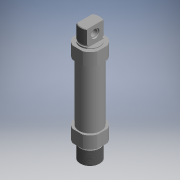
# Autodesk Inventor part: 193992 DSNU-32-60-PPS---(A----0-ZR)
Saved by Autodesk Inventor 2017.3 (Build 213256000, 256)
## iProperties
Part Number: 193992 DSNU-32-60-PPS---(A----0-ZR)
Material: Generic
Catalog Web Link: www.cadenas.de
Description: DSNU---(ZR)-Standard cylinder
Vendor: FESTO
Document SubType Name: Modeling
Designer: partserver
Manufacturer: FESTO
Mass: 95.0969 g
Surface Area: 336.432 cm^2
Volume: 95.0969 cm^3
Density: 1 g/cm^3
Appearance: PSOLRGB-192-192-192
Category: PARTsolutions
Company: FESTO
Title: 193992 DSNU-32-60-PPS
Author: Cadenas PARTsolutions
Comments: Standard cylinder
PSOL_IDENT_0: {$CADENAS_DATA\23d-libs\festo\parts\d\dsnu\parts\dsnu_metric_zr.prj},238 {VTYP=3D},{NB=193992 DSNU-3
PSOL_IDENT_1: 2-60-PPS---(A----0-ZR)},{LINA=193992 DSNU-32-60-PPS},{NN=DSNU---(ZR)},{DATE=25.01.2021 09:43:10},{GE
PSOL_IDENT_2: OMDATE=15.09.2020 12:46:13},{VERSION=},{LINEID=70},{WBVAR=TNR,HUB,DA,PE,ZD,VS,KA,K8,KP,R8},{WBNUMERI
PSOL_IDENT_3: C=HUB,K8}  {NB=193992 DSNU-32-60-PPS---(A----0-ZR)},{LINA=193992 DSNU-32-60-PPS},{KT=DUMMY},{TNR=193
PSOL_IDENT_4: 992},{TYP=DSNU-32},{DSNU=METRIC},{DE=D},{KDM=32},{HUB=60},{DA=PPS},{DA1='P','PPV','PPS'},{PE=A},{ZD=
PSOL_IDENT_5: -},{VS=-},{VSALG='-','Q'},{KA=-},{KAALG='-','S2'},{K8=0},{KP=-},{KPALG='-','KP'},{R8=-},{R81='-','R8'
PSOL_IDENT_6: },{R8H=26.200},{A1=35},{A2=500},{A3=8},{A4=55.5},{AB=30},{AM=22},{B=30},{BB=4},{BE=M30x1,5},{BENDM=3
PSOL_IDENT_7: 0.000},{BEKDM=28.160},{BEP=1.500},{BS=6.6},{B1=48},{B2=10},{B3=30},{B4=9},{B5=25.0},{B6=11},{B7=3},{
PSOL_IDENT_8: CD=10},{D=38},{D1=30},{D2=12},{D3=33.6},{D4=10.0},{D5=34.0},{D6=42},{D7=30},{EE=G1/8},{EENDM=9.7280}
PSOL_IDENT_9: ,{EEKDM=8.5660},{EW=16},{F=38},{FF=M5},{FFNDM=5.000},{FFKDM=4.019},{F1=19},{H=40},{H1=6},{KK=M10x1.2
PSOL_IDENT_10: 5},{KKNDM=10.0000},{KKKDM=8.1600},{KKP=1.250},{K1=M6},{K1NDM=6.000},{K1KDM=4.773},{K2=2.5},{KV=0},{K
PSOL_IDENT_11: W=8},{L=13},{LH=12.0},{LK=15.0},{L1=129.5},{L2=69.5},{L3=9.0},{L4=26.0},{L5=24},{L6=56},{L7=30},{L8=
PSOL_IDENT_12: 19.0},{L9=25.0},{L10=85.5},{L11=97.5},{L12=65.5},{L13=137.5},{ST=6.8},{SW=10},{T=12},{WH=34},{X=2.6}
PSOL_IDENT_13: ,{XC=117.5},{K1KP=46},{K2KP=M5},{K2KPNDM=5.000},{K3KP=12},{K4KP=23.0},{K5KP=67.5},{K6KP=4.4},{K7KP=2
PSOL_IDENT_14: 0},{K8KP=30.0},{K9KP=12.5},{K10KP=5.0},{K11KP=15},{K12KP=M5},{K12KPNDM=5.000},{K13KP=55},{ZRSTART=45
PSOL_IDENT_15: },{MHL=35.000},{ZRL=31.5},{C=17.200},{WHX=12.000},{LD1=27.800},{LD2=27.700},{AD1=11.000},{AD2=8.000}
PSOL_IDENT_16: ,{AD3=8.500},{AD4=7.000},{AD5=10.500},{MH1=11.000},{MH2=2.100},{MH3=15.200},{KP1=25.000},{KP2=26.000
PSOL_IDENT_17: },{KP3=20.000},{KP4=20.000},{KP5=36.000},{KPC=18.000},{KPF=3.000},{KPG=17.500},{KPH=62.000},{KPJ=19.
PSOL_IDENT_18: 500},{KPK=17.000},{KPL=4.500},{KPR3=1.000},{KPR=19.000},{KPS=16.000},{MLD1=45.000},{MLD2=40.000},{ML
PSOL_IDENT_19: D3=5.000},{MLL1=14.000},{PPVSTD=14.500},{PPVMH=28.000},{PPVMQ=4.500},{PPVY=9.000},{PPVZ=12.800},{PPV
PSOL_IDENT_20: A=4.000},{PPVB=0.500},{PPVC=1.000},{PPVD=1.000},{PPVE=8.000},{PPVH=15.000},{KL1=65},{SWL=6.000},{K3L=
PSOL_IDENT_21: 6.400},{ES1=2.500},{ES2=8.500},{KPVERS=0},{HUB1=60},{NUTOFF=8.500},{DIMZJREAR=181.5},{KAVERS=0},{VER
PSOL_IDENT_22: S=2},{H2=38}
NB: 193992 DSNU-32-60-PPS---(A----0-ZR)
NN: DSNU---(ZR)
NT: Standard cylinder
NBSYN: $TNR. $TYP.-$HUB1.-$DA.---($PE.$ZD.$VS.$KA.$KP.$K8.$R8.ZR)
LINA: 193992 DSNU-32-60-PPS
CATALOG: Festo
TNR: 193992
TYP: DSNU-32
DSNU: METRIC
DE: D
KDM: 32
HUB: 60
DA: PPS
DA1: 'P','PPV','PPS'
PE: A
ZD: -
VS: -
KA: -
K8: 0
KP: -
R8: -
R81: '-','R8'
R8H: 26.2
A1: 35
A2: 500
A3: 8
A4: 55.5
AB: 30
AM: 22
B: 30
BB: 4
BE: M30x1,5
BENDM: 30
BEKDM: 28.16
BEP: 1.5
BS: 6.6
B1: 48
B2: 10
B3: 30
B4: 9
B5: 25
B6: 11
B7: 3
CD: 10
D: 38
D1: 30
D2: 12
D3: 33.6
D4: 10
D5: 34
D6: 42
D7: 30
EE: G1/8
EENDM: 9.728
EEKDM: 8.566
EW: 16
F: 38
FF: M5
FFNDM: 5
FFKDM: 4.019
F1: 19
H: 40
H1: 6
KK: M10x1.25
KKNDM: 10
KKKDM: 8.16
KKP: 1.25
K1: M6
K1NDM: 6
K1KDM: 4.773
K2: 2.5
KV: 0
KW: 8
L: 13
LH: 12
LK: 15
L3: 9
L4: 26
L5: 24
L6: 56
L7: 30
L8: 19
L9: 25
L13: 137.5
ST: 6.8
SW: 10
T: 12
X: 2.6
K1KP: 46
K2KP: M5
K2KPNDM: 5
K3KP: 12
K4KP: 23
K5KP: 67.5
K6KP: 4.4
K7KP: 20
K8KP: 30
K9KP: 12.5
K10KP: 5
K11KP: 15
K12KP: M5
K12KPNDM: 5
K13KP: 55
MHL: 35
C: 17.2
WHX: 12
LD1: 27.8
LD2: 27.7
AD1: 11
AD2: 8
AD3: 8.5
AD4: 7
AD5: 10.5
MH1: 11
MH2: 2.1
MH3: 15.2
KP1: 25
KP2: 26
KP3: 20
KP4: 20
KP5: 36
KPC: 18
KPF: 3
KPG: 17.5
KPH: 62
KPJ: 19.5
KPK: 17
KPL: 4.5
KPR3: 1
KPR: 19
KPS: 16
MLD1: 45
MLD2: 40
MLD3: 5
MLL1: 14
PPVSTD: 14.5
PPVMH: 28
PPVMQ: 4.5
PPVY: 9
PPVZ: 12.8
PPVA: 4
PPVB: 0.5
PPVC: 1
PPVD: 1
PPVE: 8
PPVH: 15
SWL: 6
K3L: 6.4
ES1: 2.5
ES2: 8.5
NUTOFF: 8.5
H2: 38
SUPPLIER: FESTO
ARTICLENO: 193992 DSNU-32-60-PPS---(A----0-ZR)
BOMINFO: 193992 DSNU-32-60-PPS
CREATOR: CADENAS GmbH
Autodesk Inventor part; units mm, degrees
sketch "Sketch_12" plane through (0, 0, 0) normal (1, 0, 0) x (0, 1, 0)
  line L0 (0, -181.5) -> (0, 0)
  line L1 (0, 0) -> (14.08, 0)
  line L2 (14.08, 0) -> (15, -0.92)
  line L3 (15, -0.92) -> (15, -20.95)
  line L4 (15, -20.95) -> (14.0843, -21.8657)
  arc A0 (14.0843, -21.8657) -> (13.85, -22.4314) centre (14.65, -22.4314) ccw
  line L5 (13.85, -22.4314) -> (13.85, -23.2)
  arc A1 (13.85, -23.2) -> (14.65, -24) centre (14.65, -23.2) ccw
  line L6 (14.65, -24) -> (15, -24)
  line L7 (15, -24) -> (15, -26.1)
  line L8 (15, -26.1) -> (20.5, -26.1)
  line L9 (20.5, -26.1) -> (20.5, -45.05)
  line L10 (20.5, -45.05) -> (16.8, -45.05)
  line L11 (16.8, -45.05) -> (16.8, -136.45)
  line L12 (16.8, -136.45) -> (20.5, -136.45)
  line L13 (20.5, -136.45) -> (20.5, -155.4)
  line L14 (20.5, -155.4) -> (15, -155.4)
  line L15 (15, -155.4) -> (15, -157.5)
  line L16 (15, -157.5) -> (14.65, -157.5)
  arc A2 (14.65, -157.5) -> (13.85, -158.3) centre (14.65, -158.3) ccw
  line L17 (13.85, -158.3) -> (13.85, -159.0686)
  arc A3 (13.85, -159.0686) -> (14.0843, -159.6343) centre (14.65, -159.0686) ccw
  line L18 (14.0843, -159.6343) -> (15, -160.55)
  line L19 (15, -160.55) -> (15, -180.58)
  line L20 (15, -180.58) -> (14.08, -181.5)
  line L21 (14.08, -181.5) -> (0, -181.5)
  line L22 (0, -181.5) -> (0, 0)
  constraints: 46 end point, 8 point on circle, 4 centre point
revolve "Revolution1" add sketch "Sketch_12" angle 360 about axis through (0, 0, -181.5) along (0, 0, -1)
thread "Thread1" size "M30x1.5" class "6g" standard "ISO Metric profile" full length
thread "Thread2" size "M30x1.5" class "6g" standard "ISO Metric profile" full length
sketch "Sketch_1" plane through (0, 0, 0) normal (0, 0, 1) x (1, 0, 0)
  line L0 (-38, 38) -> (-38, -38)
  line L1 (-38, -38) -> (38, -38)
  line L2 (38, -38) -> (38, 38)
  line L3 (38, 38) -> (-38, 38)
  line L4 (-19, 19) -> (-19, -19)
  line L5 (-19, -19) -> (19, -19)
  line L6 (19, -19) -> (19, 19)
  line L7 (19, 19) -> (-19, 19)
  constraints: 16 end point
extrude "Extrusion1" cut sketch "Sketch_1" against normal blind 189.5
sketch "Sketch_124" plane through (0, 0, 0) normal (0, 1, 0) x (-1, 0, 0)
  line L0 (38, -156.5) -> (8, -156.5)
  line L1 (8, -156.5) -> (8, -181.5)
  line L2 (8, -181.5) -> (-8, -181.5)
  line L3 (-8, -181.5) -> (-8, -156.5)
  line L4 (-8, -156.5) -> (-38, -156.5)
  line L5 (-38, -156.5) -> (-38, -186.5)
  line L6 (-38, -186.5) -> (38, -186.5)
  line L7 (38, -186.5) -> (38, -156.5)
  constraints: 16 end point
extrude "Extrusion2" cut sketch "Sketch_124" along normal mid plane 38
sketch "Sketch_3" plane through (0, 0, -169.5) normal (0, 0, 1) x (1, 0, 0)
  line L0 (8, 0) -> (-8, 0)
  line L1 (-8, 0) -> (-8, 6.5774)
  line L2 (-8, 6.5774) -> (-7, 6)
  line L3 (-7, 6) -> (-6, 6)
  line L4 (-6, 6) -> (-6, 5)
  line L5 (-6, 5) -> (6, 5)
  line L6 (6, 5) -> (6, 6)
  line L7 (6, 6) -> (7, 6)
  line L8 (7, 6) -> (8, 6.5774)
  line L9 (8, 6.5774) -> (8, 0)
  line L10 (8, 0) -> (-8, 0)
  constraints: 22 end point
revolve "Revolution2" cut sketch "Sketch_3" angle 360 about axis through (8, 0, -169.5) along (1, 0, 0)
sketch "Sketch5" plane through (-7.6974, 19, -26.1) normal (0, 1, 0) x (1, 0, 0)
  point P0 (7.6974, 9)
hole "Hole1" at (0, 19, -35.1) direction (0, -1, 0) diameter 8.566 depth 19 countersink diameter 9.728 countersink angle 90 thread size "G9.728x0.907" designation "G 1/8" standard "ISO Pipe Threads"
sketch "Sketch6" plane through (-7.6974, 19, -136.45) normal (0, 1, 0) x (1, 0, 0)
  point P0 (7.6974, 9.95)
hole "Hole2" at (0, 19, -146.4) direction (0, -1, 0) diameter 8.566 depth 8.5 tip angle 120 countersink diameter 9.728 countersink angle 90 thread size "G9.728x0.907" designation "G 1/8" standard "ISO Pipe Threads"
sketch "Sketch_129" plane through (0, 0, 0) normal (1, 0, 0) x (0, 1, 0)
  line L0 (0, -125) -> (0, 8)
  line L1 (0, 8) -> (6, 8)
  line L2 (6, 8) -> (6, -57)
  line L3 (6, -57) -> (16, -57)
  line L4 (16, -57) -> (16, -125)
  line L5 (16, -125) -> (0, -125)
  line L6 (0, -125) -> (0, 8)
  constraints: 14 end point
revolve "Revolution3" cut sketch "Sketch_129" angle 360 about axis through (0, 0, -125) along (0, 0, -1)
ref_plane "FDT_FRONT_XY" through (0, 0, -26.1) normal (0, 0, -1) x (1, 0, 0)
ref_plane "FDT_FRONT_YZ" through (0, 0, -26.1) normal (1, 0, 0) x (0, -1, 0)
ref_plane "FDT_FRONT_ZX" through (0, 0, -26.1) normal (0, -1, 0) x (0, 0, -1)
ref_plane "FDT_QSFRONT_XY" through (0, 19, -35.1) normal (0, 1, 0) x (0, 0, 1)
ref_plane "FDT_QSFRONT_YZ" through (0, 19, -35.1) normal (0, 0, 1) x (1, 0, 0)
ref_plane "FDT_QSFRONT_ZX" through (0, 19, -35.1) normal (1, 0, 0) x (0, 1, 0)
ref_plane "FDT_QSREAR_XY" through (0, 19, -146.4) normal (0, 1, 0) x (0, 0, 1)
ref_plane "FDT_QSREAR_YZ" through (0, 19, -146.4) normal (0, 0, 1) x (1, 0, 0)
ref_plane "FDT_QSREAR_ZX" through (0, 19, -146.4) normal (1, 0, 0) x (0, 1, 0)
ref_plane "FDT_REAR_XY" through (0, 0, -155.4) normal (0, 0, 1) x (1, 0, 0)
ref_plane "FDT_REAR_YZ" through (0, 0, -155.4) normal (1, 0, 0) x (0, 1, 0)
ref_plane "FDT_REAR_ZX" through (0, 0, -155.4) normal (0, 1, 0) x (0, 0, 1)
ref_plane "FDT_SMBR1_XY" through (0, 0, -54.5) normal (0, 0, 1) x (-1, 0, 0)
ref_plane "FDT_SMBR1_YZ" through (0, 0, -54.5) normal (-1, 0, 0) x (0, -1, 0)
ref_plane "FDT_SMBR1_ZX" through (0, 0, -54.5) normal (0, -1, 0) x (0, 0, 1)
ref_plane "FDT_SMBR2_XY" through (0, 0, -127) normal (0, 0, 1) x (-1, 0, 0)
ref_plane "FDT_SMBR2_YZ" through (0, 0, -127) normal (-1, 0, 0) x (0, -1, 0)
ref_plane "FDT_SMBR2_ZX" through (0, 0, -127) normal (0, -1, 0) x (0, 0, 1)
ref_plane "FDT_SWIVELAXIS_XY" through (0, 0, -169.5) normal (1, 0, 0) x (0, 0, -1)
ref_plane "FDT_SWIVELAXIS_YZ" through (0, 0, -169.5) normal (0, 0, -1) x (0, 1, 0)
ref_plane "FDT_SWIVELAXIS_ZX" through (0, 0, -169.5) normal (0, 1, 0) x (1, 0, 0)
ref_plane "NUT_XY" through (0, 0, -8.5) normal (0, 0, -1) x (1, 0, 0)
ref_plane "NUT_YZ" through (0, 0, -8.5) normal (1, 0, 0) x (0, -1, 0)
ref_plane "NUT_ZX" through (0, 0, -8.5) normal (0, -1, 0) x (0, 0, -1)
ref_plane "ZR_XY" through (0, 0, 0) normal (0, 0, -1) x (-1, 0, 0)
ref_plane "ZR_YZ" through (0, 0, 0) normal (-1, 0, 0) x (0, 1, 0)
ref_plane "ZR_ZX" through (0, 0, 0) normal (0, 1, 0) x (0, 0, -1)
ref_plane "ZYL_XY" through (0, 0, -26.1) normal (0, 0, -1) x (1, 0, 0)
ref_plane "ZYL_YZ" through (0, 0, -26.1) normal (1, 0, 0) x (0, -1, 0)
ref_plane "ZYL_ZX" through (0, 0, -26.1) normal (0, -1, 0) x (0, 0, -1)
body "Solid1"
